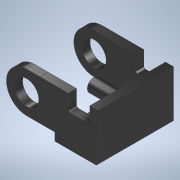
# Autodesk Inventor part: X-linear bearing shroud-A(original)
Saved by Autodesk Inventor 2020.4 (Build 244396000, 396)
## iProperties
Created: 2021-02-25
Part Number: X-linear bearing shroud-A(original)
Material: ABS Plastic
Document SubType Name: Modeling
Designer: AOB
Mass: 5.0913 g
Surface Area: 40.0439 cm^2
Volume: 4.80311 cm^3
Density: 1.06 g/cm^3
Appearance: Glossy - Black
Author: AOB
Autodesk Inventor part; units mm, degrees
ref_plane "YZ Plane" through (0, 0, 0) normal (1, 0, 0) x (0, 1, 0)
ref_plane "XZ Plane" through (0, 0, 0) normal (0, 1, 0) x (-1, 0, 0)
sketch "Sketch1" plane through (0, 0, 0) normal (0, 0, 1) x (1, 0, 0)
  line L0 (5.0224, 7.5) -> (15.5, 7.5)
  line L1 (5.0224, 7.5) -> (5.7962, 7.5)
  arc A0 (0, 7.5) -> (-0.0125, -7.5) centre (0, 0) ccw
  line L2 (5.0224, 7.5) -> (0, 7.5)
  line L3 (-0.0125, -7.5) -> (10.4785, -7.5)
  line L4 (21.9991, -10.4606) -> (10.4785, -10.4606)
  line L5 (10.4785, -10.4606) -> (10.4785, -7.5)
  line L6 (16, 1.4713) -> (23, 1.4713)
  line L7 (23.5, 1.9713) -> (23.5, 7.5001)
  line L8 (23.5, 7.5001) -> (26.5, 7.5001)
  line L9 (26.5, 7.5001) -> (26.5, -9.4606)
  line L10 (25.5, -10.4606) -> (21.9991, -10.4606)
  arc A1 (25.5, -10.4606) -> (26.5, -9.4606) centre (25.5, -9.4606) ccw
  line L11 (23, 1.4713) -> (23.5, 1.9713)
  line L12 (15.5, 7.5001) -> (15.5, 1.9713)
  line L13 (16, 1.4713) -> (15.5, 1.9713)
  point P0 (23.5, 1.4713)
  point P1 (15.5, 1.4713)
  dimension "d47" = 10.491
  dimension "d57" = 3
  dimension "d58" = 1
  dimension "d62" = 8
  dimension "d65" = 15.5
  constraints: 28 end point, 6 point on line, 4 horizontal, 4 perpendicular, 4 point on circle, 3 tangent, 2 centre point, 1 coincident, 1 vertical
  measures "d47" distance of L3.start L3.end
  measures "d57" distance of L7.end L8.end
  measures "d58" radius of A1
  measures "d62" distance of L7.end L12.start
  measures "d65" distance from line of point (0, 0) L12
extrude "Extrusion1" add sketch "Sketch1" along normal blind 3
sketch "Sketch3" plane through (0, 0, 0) normal (0, 0, -1) x (-1, 0, 0)
  line L0 (-20.0398, -7.5) -> (-10.4968, -7.5)
  line L1 (-10.4968, -7.5) -> (-10.4968, -7.5)
  line L2 (-26.5, -9.4606) -> (-26.5, 7.5001) projected
  line L3 (-26.5, 7.5001) -> (-23.5, 7.5001) projected
  line L4 (-23.5, 7.5001) -> (-23.5, 1.9713) projected
  line L5 (-10.4785, -10.4606) -> (-25.5, -10.4606) projected
  arc A0 (-26.5, -9.4606) -> (-25.5, -10.4606) centre (-25.5, -9.4606) ccw projected
  line L6 (-23.5, 1.9713) -> (-23.5, -7.5)
  line L7 (-23.5, -7.5) -> (-20.0398, -7.5)
  line L8 (-10.4785, -7.5) -> (-10.4785, -10.4606) projected
  dimension "d44" = 9.543
  constraints: 8 end point, 1 perpendicular, 1 vertical
  measures "d44" distance of L1.start L0.start
extrude "Extrusion3" add sketch "Sketch3" along normal blind 11 fills toward (-10.5285, -8.9803) open curves L8 L5 A0 L2 L3 L4 L6 L7 L0 L1
ref_plane "Work Plane1" through (0, 0, -11) normal (0, 0, -1) x (-1, 0, 0)
sketch "Sketch4" plane through (23.5, 6.9501, 0) normal (-1, 0, 0) x (0, 0, 1)
  circle A0 centre (-11, -6) radius 2.5
  point P0 (0, -6.9501)
  dimension "d22" = 5
  constraints: 1 centre point
  measures "d22" diameter of A0
extrude "Extrusion4" add sketch "Sketch4" along normal blind 12.5
sketch "Sketch6" plane through (0, 0, 0) normal (0, 0, -1) x (-1, 0, 0)
  arc A0 (-5.0224, 5.57) -> (0, 7.5) centre (0, 0) ccw
  arc A1 (5.0224, 5.5902) -> (0, 7.5) centre (0, -0.0589) ccw
  line L0 (-5.0224, 5.57) -> (-5.0224, 7.5)
  line L1 (-5.0224, 7.5) -> (-5.0224, 5.57)
  line L2 (-5.0224, 7.5) -> (0, 7.5) projected
  line L3 (-5.0224, 7.5) -> (0, 7.5)
  circle A2 centre (0, -0.0589) radius 4.5
  point P0 (5.0224, 5.5902)
  dimension "d37" = 9
  constraints: 6 end point, 4 point on circle, 3 centre point, 2 coincident, 2 collinear, 1 tangent, 1 vertical
  measures "d37" diameter of A2
extrude "Extrusion8" [suppressed]
extrude "Extrusion9" cut sketch "Sketch6" against normal through all contours A2
mirror "Mirror4" about plane through (0, 0, -11) normal (0, 0, -1) of "Extrusion1", "Extrusion3", "Extrusion9"
sketch "Sketch7" plane through (23.034, -9.4606, 0) normal (0.9999999, -0.0004249, 0) x (0, 0, -1)
  line L0 (0, -1.0053) -> (22, -1.0053) projected
  circle A0 centre (11, 3.4947) radius 4
  point P0 (0, 9.4508)
  dimension "d49" = 8
  constraints: 1 centre point
  measures "d49" diameter of A0
extrude "Extrusion10" [suppressed]
body "Solid1"
